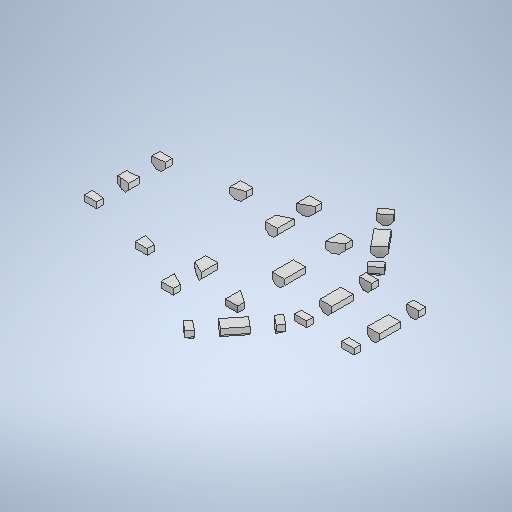
# Autodesk Inventor part: RR_SingleTurnout_Pillow
Saved by Autodesk Inventor 2025.1 (Build 291241000, 241)
## iProperties
Created: 2025-03-08
Part Number: RR_SingleTurnout_Pillow
Material: 一般
Document SubType Name: Modeling
Designer: kumagai
Density: 1 g/cm^3
Appearance: 既定
Author: kumagai
Autodesk Inventor part; units mm, degrees
ref_plane "YZ Plane" through (0, 0, 0) normal (1, 0, 0) x (0, 1, 0)
ref_plane "XZ Plane" through (0, 0, 0) normal (0, 1, 0) x (-1, 0, 0)
ref_plane "XY Plane" through (0, 0, 0) normal (0, 0, 1) x (1, 0, 0)
derived "RR_ThreeWay.ipt"
sketch "MainSketch" plane through (0, 0, 0) normal (0, 1, 0) x (-1, 0, 0)
  line L0 (0, -344.2613) -> (0, 286.2613)
  line L1 (-272.9287, 0) -> (62.5724, 0)
  line L2 (14.6437, -29) -> (-5, -29)
  line L3 (-5, -49.5106) -> (-5, -5.6416)
  line L4 (-5, -48) -> (0, -48)
  line L5 (-5, -10) -> (0, -10)
  line L6 (-5, -38.3) -> (0, -38.3)
  line L7 (-5, -19.7) -> (0, -19.7)
  line L8 (-5, -46) -> (0, -46)
  line L9 (-5, -35.9) -> (0, -35.9)
  line L10 (-5, -22.1) -> (0, -22.1)
  line L11 (-5, -12) -> (0, -12)
  line L12 (-10, -10) -> (-10, -29)
  line L13 (-225, -48) -> (-225, -29)
  line L14 (-120.9077, -19.7) -> (-225, -19.7)
  arc A0 (-10, -48) -> (-148.5929, -105.4071) centre (-10, -244) ccw
  arc A1 (-10, -46) -> (-150.0071, -103.9929) centre (-10, -244) ccw
  line L15 (-143.2215, -110.7785) -> (-189.5102, -64.4898)
  line L16 (-210, -35.9) -> (-210, -29)
  line L17 (-146.1596, -86.6272) -> (-155.9415, -76.8453)
  arc A2 (-133.8847, -47.8455) -> (-174.0488, -79.9512) centre (-10, -244) ccw
  arc A3 (-139.2229, -48.9168) -> (-175.463, -78.537) centre (-10, -244) ccw
  line L18 (-139.499, -48) -> (-225, -48)
  line L19 (-134.4186, -46) -> (-225, -46)
  arc A4 (-118.9103, -50.6657) -> (-166.907, -87.093) centre (-10, -244) ccw
  arc A5 (-120.0882, -48.5746) -> (-168.6041, -85.3959) centre (-10, -244) ccw
  line L20 (-94.2219, -46) -> (-110.2721, -46)
  arc A6 (-111.9271, -35.5897) -> (-114.1724, -36.7028) centre (-10, -244) ccw
  line L21 (-120.9077, -35.9) -> (-225, -35.9)
  line L22 (-120.9077, -38.3) -> (-225, -38.3)
  arc A7 (-133.8847, -47.8455) -> (-134.4186, -46) centre (-134.4186, -47) ccw
  arc A8 (-139.2229, -48.9168) -> (-139.499, -48) centre (-139.499, -48.5) ccw
  arc A9 (-110.2721, -48.4) -> (-118.9103, -50.6657) centre (-110.2721, -66) ccw
  arc A10 (-110.2721, -46) -> (-120.0882, -48.5746) centre (-110.2721, -66) ccw
  arc A11 (-120.9077, -38.3) -> (-114.1724, -36.7028) centre (-120.9077, -23.3) ccw
  arc A12 (-120.9077, -35.9) -> (-115.25, -34.5584) centre (-120.9077, -23.3) ccw
  arc A13 (-143.5264, -51.2283) -> (-148.5252, -54.7884) centre (-10, -244) ccw
  arc A14 (-112.9815, -33.4337) -> (-115.25, -34.5584) centre (-10, -244) ccw
  line L23 (-120.9077, -22.1) -> (-225, -22.1)
  circle A15 centre (-86.125, -22.2) radius 2.5
  arc A16 (-96.415, -52.9331) -> (-105.3417, -57.2273) centre (-10, -244) ccw
  arc A17 (-96.4922, -49.4759) -> (-95.7188, -53.2122) centre (-89.6121, -50) ccw
  arc A18 (-93.3838, -47.5455) -> (-92.1285, -53.7307) centre (-89.6121, -50) ccw
  arc A19 (-96.1897, -54.5879) -> (-157.1489, -96.8511) centre (-10, -244) ccw
  line L24 (-97.4893, -48.4) -> (-110.2721, -48.4)
  arc A20 (-92.2877, -55.4762) -> (-155.4519, -98.5481) centre (-10, -244) ccw
  arc A21 (-92.2877, -55.4762) -> (-92.1285, -53.7307) centre (-92.6877, -54.5597) ccw
  arc A22 (-93.3838, -47.5455) -> (-94.2219, -46) centre (-94.2219, -47) ccw
  arc A23 (-96.1897, -54.5879) -> (-95.7188, -53.2122) centre (-96.6039, -53.6777) ccw
  arc A24 (-96.4922, -49.4759) -> (-97.4893, -48.4) centre (-97.4893, -49.4) ccw
  circle A25 centre (-89.6121, -50) radius 2.5
  line L25 (-42.4799, -17.7596) -> (-25.8571, -19.9879)
  arc A26 (-25.9153, -20.5847) -> (-85.6348, -24.6515) centre (-40.1446, -252.1479) ccw
  arc A27 (-85.7928, -19.7222) -> (-85.6348, -24.6515) centre (-86.125, -22.2) ccw
  arc A28 (-25.9153, -20.5847) -> (-25.8571, -19.9879) centre (-25.8969, -20.2853) ccw
  arc A29 (-42.4799, -17.7596) -> (-76.3848, -20.5664) centre (-40.1446, -252.1479) ccw
  line L26 (-85.7928, -19.7222) -> (-79.2595, -20.598)
  arc A30 (-79.2595, -20.598) -> (-76.3848, -20.5664) centre (-77.9308, -10.6866) ccw
  circle A31 centre (-89.6121, -50) radius 4
  line L27 (-89.754, -46.0025) -> (-25.5965, -43.7259)
  arc A32 (-25.552, -44.3238) -> (-40.8225, -46.6677) centre (-3.1703, -241.0547) ccw
  arc A33 (-25.552, -44.3238) -> (-25.5965, -43.7259) centre (-25.5859, -44.0257) ccw
  arc A34 (-74.4895, -48.1141) -> (-87.9633, -53.6443) centre (-3.1703, -241.0547) ccw
  line L28 (-72.9332, -47.8071) -> (-40.8225, -46.6677)
  arc A35 (-72.9332, -47.8071) -> (-74.4895, -48.1141) centre (-72.7559, -52.804) ccw
  arc A36 (-44.0479, -18.9806) -> (-84.6326, -23.2308) centre (-40.1446, -252.1479) ccw
  arc A37 (-27.9859, -39.0878) -> (-44.4613, -41.2072) centre (-10, -244) ccw
  line L29 (-31.1334, -19.7) -> (-47.6548, -19.7)
  arc A38 (-10, -22.1) -> (-22.0271, -22.4262) centre (-10, -244) ccw
  arc A39 (-44.7432, -24.8368) -> (-62.9678, -28.5145) centre (-10, -244) ccw
  arc A40 (-10, -19.7) -> (-22.1572, -20.0297) centre (-10, -244) ccw
  arc A41 (-45.119, -22.4664) -> (-72.2793, -28.5197) centre (-10, -244) ccw
  arc A42 (-25.457, -23.6967) -> (-43.178, -22.3501) centre (-51.8841, -254.1867) ccw
  line L30 (-24.9, -22.9254) -> (-24.9, -23.2)
  arc A43 (-25.457, -23.6967) -> (-24.9, -23.2) centre (-25.4, -23.2) ccw
  arc A44 (-22.1572, -20.0297) -> (-24.9, -22.9254) centre (-22, -22.9254) ccw
  arc A45 (-43.178, -22.3501) -> (-45.119, -22.4664) centre (-43.5532, -32.343) ccw
  arc A46 (-25.7303, -26.0811) -> (-43.268, -24.7484) centre (-51.8841, -254.1867) ccw
  arc A47 (-22.0271, -22.4262) -> (-22.5, -22.9254) centre (-22, -22.9254) ccw
  line L31 (-22.5, -22.9254) -> (-22.5, -23.2)
  arc A48 (-25.7303, -26.0811) -> (-22.5, -23.2) centre (-25.4, -23.2) ccw
  arc A49 (-43.268, -24.7484) -> (-44.7432, -24.8368) centre (-43.5532, -32.343) ccw
  line L32 (-55.2, -53.283) -> (-55.2, -10)
  line L33 (-40.8, -50.4351) -> (-40.8, -10)
  line L34 (-48, 3.552) -> (-48, 5.2256)
  line L35 (-59, -61.5) -> (-37, -61.5)
  line L36 (-40.8, -10) -> (-40.8, -7.4996)
  line L37 (-55.2, -10) -> (-55.2, -7.4996)
  line L38 (-48, -61.9179) -> (-48, -64.1825)
  line L39 (-37, -61.5) -> (-37, -70.5)
  line L40 (-40, -73.5) -> (-42, -73.5)
  line L41 (-42, -73.5) -> (-40, -62)
  line L42 (-40, -62) -> (-56, -62)
  line L43 (-56, -62) -> (-54, -73.5)
  line L44 (-54, -73.5) -> (-56, -73.5)
  line L45 (-59, -70.5) -> (-59, -58.1371)
  arc A50 (-40, -73.5) -> (-37, -70.5) centre (-40, -70.5) ccw
  arc A51 (-59, -70.5) -> (-56, -73.5) centre (-56, -70.5) ccw
  line L46 (-37, -61.5) -> (-37, -49.8686)
  line L47 (-40.8, -50.4351) -> (-40.8, -62)
  line L48 (-55.2, -53.283) -> (-55.2, -62)
  arc A52 (-34.3731, -49.5213) -> (-37, -52.498) centre (-34, -52.498) ccw
  arc A53 (-59, -58.1371) -> (-62.8083, -55.2481) centre (-62, -58.1371) ccw
  line L49 (-10, -29) -> (-225, -29)
  arc A54 (-151.7465, 120.5538) -> (-11.4945, 29.8813) centre (-10, 186) ccw
  arc A55 (-22.0271, -35.5738) -> (-10, -35.9) centre (-10, 186) ccw
  arc A56 (-22.1572, -37.9703) -> (-10, -38.3) centre (-10, 186) ccw
  arc A57 (-43.268, -33.2516) -> (-25.7303, -31.9189) centre (-51.8841, 196.1867) ccw
  arc A58 (-43.178, -35.6499) -> (-25.457, -34.3033) centre (-51.8841, 196.1867) ccw
  arc A59 (-62.9678, -29.4855) -> (-44.7432, -33.1632) centre (-10, 186) ccw
  arc A60 (-72.2793, -29.4803) -> (-45.119, -35.5336) centre (-10, 186) ccw
  arc A61 (-45.119, -35.5336) -> (-43.178, -35.6499) centre (-43.5532, -25.657) ccw
  arc A62 (-44.7432, -33.1632) -> (-43.268, -33.2516) centre (-43.5532, -25.657) ccw
  arc A63 (-22.5, -35.0746) -> (-22.0271, -35.5738) centre (-22, -35.0746) ccw
  arc A64 (-24.9, -35.0746) -> (-22.1572, -37.9703) centre (-22, -35.0746) ccw
  line L50 (-24.9, -35.0746) -> (-24.9, -34.8)
  line L51 (-22.5, -35.0746) -> (-22.5, -34.8)
  arc A65 (-24.9, -34.8) -> (-25.457, -34.3033) centre (-25.4, -34.8) ccw
  arc A66 (-22.5, -34.8) -> (-25.7303, -31.9189) centre (-25.4, -34.8) ccw
  arc A67 (-62.9678, -28.5145) -> (-63.3485, -29) centre (-62.8485, -29) ccw
  arc A68 (-72.2793, -28.5197) -> (-72.6405, -29) centre (-72.1405, -29) ccw
  arc A69 (-108.1902, -15.666) -> (-89.3785, -23.7845) centre (-10, 186) ccw
  arc A70 (-91.0057, 5.3288) -> (-16.6975, -11.8867) centre (-10, 186) ccw
  arc A71 (-122.8924, 131.193) -> (-43.8763, 65.1658) centre (-10, 186) ccw
  arc A72 (-148.5252, -3.2116) -> (-143.5264, -6.7717) centre (-10, 186) ccw
  circle A73 centre (-86.125, -35.8) radius 2.5
  arc A74 (-85.7286, -33.3316) -> (-25.8975, -35.1189) centre (-48.9436, 195.7336) ccw
  line L52 (-25.8166, -35.7131) -> (-42.3424, -38.5735)
  arc A75 (-25.8166, -35.7131) -> (-25.8975, -35.1189) centre (-25.8677, -35.4174) ccw
  line L53 (-85.6986, -38.2634) -> (-79.2034, -37.1391)
  arc A76 (-76.3296, -37.0611) -> (-79.2034, -37.1391) centre (-77.4979, -46.9926) ccw
  arc A77 (-76.3296, -37.0611) -> (-42.3424, -38.5735) centre (-48.9436, 195.7336) ccw
  arc A78 (-49.1227, -37.4664) -> (-46.0444, -37.4484) centre (-48.9436, 195.7336) ccw
  line L54 (-86.4807, -38.2746) -> (-94.1197, -37.1765)
  arc A79 (-94.2268, -36.2144) -> (-94.1197, -37.1765) centre (-94.0486, -36.6816) ccw
  line L55 (-87.0159, -33.4641) -> (-94.2268, -36.2144)
  line L56 (-76.4926, -34.8148) -> (-77.6457, -34.6296)
  arc A80 (-96.055, -36.8647) -> (-107.6082, -42.0517) centre (-10, -244) ccw
  circle A81 centre (-89.6121, -8) radius 4
  line L57 (-89.6178, -12) -> (-25.42, -12.0915)
  arc A82 (-88.0883, -4.3016) -> (-74.4341, -9.37) centre (-9.7235, 185.8863) ccw
  arc A83 (-74.4341, -9.37) -> (-72.8683, -9.6239) centre (-72.8611, -4.6239) ccw
  line L58 (-72.8683, -9.6239) -> (-40.7373, -9.6697)
  arc A84 (-40.7373, -9.6697) -> (-25.3959, -11.4925) centre (-9.7235, 185.8863) ccw
  arc A85 (-25.42, -12.0915) -> (-25.3959, -11.4925) centre (-25.4196, -11.7915) ccw
  line L59 (-41.4, -73.5) -> (-41.4, -70.05)
  line L60 (-54.6, -73.5) -> (-54.6, -70.05)
  line L61 (-21.7393, -64.7371) -> (-21.7393, -55.7371)
  line L62 (-51.6, 5.7033) -> (-51.6, 3.6437)
  line L63 (-44.4, 6.6538) -> (-44.4, 3.6437)
  line L64 (-44.4, -63.9796) -> (-44.4, -61.3243)
  line L65 (-51.6, -63.5159) -> (-51.6, -61.3243)
  arc A86 (-106.8215, -31.0506) -> (-105.9722, -29) centre (-108.8722, -29) ccw
  arc A87 (-111.9271, -35.5897) -> (-109.9456, -34.1747) centre (-115.1782, -28.9421) ccw
  line L66 (-109.9456, -34.1747) -> (-106.8215, -31.0506)
  arc A88 (-112.9815, -33.4337) -> (-111.6427, -32.4776) centre (-115.1782, -28.9421) ccw
  arc A89 (-108.5186, -29.3536) -> (-108.3722, -29) centre (-108.8722, -29) ccw
  line L67 (-111.6427, -32.4776) -> (-108.5186, -29.3536)
  arc A90 (-63.3485, -29) -> (-62.9678, -29.4855) centre (-62.8485, -29) ccw
  arc A91 (-72.6405, -29) -> (-72.2793, -29.4803) centre (-72.1405, -29) ccw
  line L68 (-210, -29) -> (-210, -22.1)
  line L69 (-225, -29) -> (-225, -10)
  line L70 (-10, -29) -> (-10, -48)
  line L71 (-22.0231, -12) -> (-39.3668, -12)
  line L72 (-157.1489, -96.8511) -> (-146.5423, -86.2445)
  point P0 (0, 0)
  point P1 (-90.8602, -19.7)
  point P2 (-94.9346, -22.1)
  point P3 (-96.3241, -48.4)
  point P4 (-87.5506, -46)
  point P5 (-162.028, -91.972)
  point P6 (-44.0258, -45.5806)
  point P7 (-48, -2.9806)
  point P8 (-48, -61.5806)
  point P9 (-37, -73.5)
  point P10 (-59, -73.5)
  point P11 (-51.2642, -37.4549)
  point P12 (-51.1178, -10.8549)
  point P13 (-103.3722, -29)
  point P14 (-48, -53.4549)
sketch "PillowSketch" plane through (0, 0, 0) normal (0, 1, 0) x (-1, 0, 0)
  line L0 (-40, -1.4534) -> (-40, 7.7945)
  line L1 (-71, -1.7421) -> (-71, 3.0229)
  line L2 (-102, -0.653) -> (-102, 5.4734)
  line L3 (-133, -1.0497) -> (-133, 3.4642)
  line L4 (-164, -2.8834) -> (-164, 3.4642)
  line L5 (-195, -2.8121) -> (-195, 3.534)
  line L6 (-121.4315, -106.3936) -> (-109.7227, -120.8528)
  line L7 (-101.8172, -89.6691) -> (-92.4243, -105.4573)
  line L8 (-79.3942, -76.4675) -> (-71.1859, -96.2843)
  line L9 (-75, -63.4919) -> (-67, -63.4919)
  line L10 (-106, -77.5199) -> (-98, -77.5199)
  line L11 (-156.8999, -56.2377) -> (-163.117, -61.2723)
  line L12 (-133.6607, -97.6478) -> (-127.4435, -92.6133)
  line L13 (-137, -66.4368) -> (-129, -66.4368)
  line L14 (-168, -52.4) -> (-160, -52.4)
  line L15 (-199, -52.4) -> (-191, -52.4)
  line L16 (-160, -52.4) -> (-160, -48)
  line L17 (-168, -48) -> (-168, -52.4)
  line L18 (-191, -52.4) -> (-191, -48)
  line L19 (-199, -48) -> (-199, -52.4)
  line L20 (-137, -62.0368) -> (-137, -66.4368)
  line L21 (-129, -66.4368) -> (-129, -56.7072)
  line L22 (-98, -77.5199) -> (-98, -68.8658)
  line L23 (-98, -55.4221) -> (-98, -48.4)
  line L24 (-106, -48.4) -> (-106, -59.3663)
  line L25 (-106, -73.1199) -> (-106, -77.5199)
  line L26 (-67, -63.4919) -> (-67, -56.4713)
  line L27 (-75, -59.0919) -> (-75, -63.4919)
  line L28 (-28, -2.7496) -> (-28, 7.3369)
  line L29 (-32, -53.6386) -> (-24, -53.6386)
  line L30 (-24, -53.6386) -> (-24, -48.5006)
  line L31 (-32, -49.2386) -> (-32, -53.6386)
  line L32 (-136.4297, -94.2284) -> (-133.6607, -97.6478)
  line L33 (-127.4435, -92.6133) -> (-130.2125, -89.1938)
  line L34 (-163.117, -61.2723) -> (-160.348, -64.6917)
  line L35 (-152.7321, -74.0966) -> (-144.046, -84.8231)
  line L36 (-137.8288, -79.7885) -> (-146.5149, -69.062)
  line L37 (-154.1309, -59.6571) -> (-156.8999, -56.2377)
  line L38 (-143.2215, -110.7785) -> (-189.5102, -64.4898) projected
  arc A0 (-10, -48) -> (-148.5929, -105.4071) centre (-10, -244) ccw projected
  arc A1 (-139.2229, -48.9168) -> (-175.463, -78.537) centre (-10, -244) ccw projected
  arc A2 (-96.1897, -54.5879) -> (-157.1489, -96.8511) centre (-10, -244) ccw projected
  arc A3 (-118.9103, -50.6657) -> (-166.907, -87.093) centre (-10, -244) ccw projected
  line L39 (-97.4893, -48.4) -> (-110.2721, -48.4) projected
  line L40 (-10, -29) -> (-225, -29) projected
  line L41 (-120.9077, -35.9) -> (-225, -35.9) projected
  line L42 (-225, -48) -> (-225, -29) projected
  line L43 (-10, -29) -> (-10, -48) projected
  line L44 (-139.499, -48) -> (-225, -48) projected
  line L45 (-160, -35.9) -> (-160, -29)
  line L46 (-168, -35.9) -> (-168, -29)
  line L47 (-191, -35.9) -> (-191, -29)
  line L48 (-199, -35.9) -> (-199, -29)
  arc A4 (-43.268, -33.2516) -> (-25.7303, -31.9189) centre (-51.8841, 196.1867) ccw projected
  arc A5 (-22.5, -34.8) -> (-25.7303, -31.9189) centre (-25.4, -34.8) ccw projected
  arc A6 (-25.7303, -26.0811) -> (-22.5, -23.2) centre (-25.4, -23.2) ccw projected
  arc A7 (-25.7303, -26.0811) -> (-43.268, -24.7484) centre (-51.8841, -254.1867) ccw projected
  line L49 (-32, -32.5507) -> (-32, -29)
  line L50 (-24, -32.6357) -> (-24, -29)
  line L51 (-129, -35.9) -> (-129, -29)
  line L52 (-137, -35.9) -> (-137, -29)
  point P0 (0, 0)
  point P1 (-24, -32.2603)
  dimension "d2" = 31
  dimension "d3" = 31
  dimension "d4" = 31
  dimension "d5" = 31
  dimension "d6" = 31
  dimension "d9" = 8.25
  dimension "d10" = 8.25
  dimension "d17" = 4.4
  dimension "d19" = 4.4
  dimension "d21" = 4.4
  dimension "d25" = 4.4
  dimension "d27" = 8
  dimension "d28" = 4.4
  dimension "d29" = 4.4
  dimension "d38" = 30
  dimension "d39" = 30
  dimension "d40" = 18
  dimension "d41" = 6
  dimension "d42" = 8
  dimension "d43" = 8
  dimension "d44" = 8
  dimension "d45" = 8
  dimension "d46" = 8
  dimension "d47" = 8
  dimension "d48" = 4.4
  constraints: 92 end point, 16 point on line, 15 collinear, 11 point on circle, 6 perpendicular, 6 vertical, 4 horizontal, 3 parallel, 25 other
  measures "d2" distance between parallel lines of L4 L5
  measures "d3" distance between parallel lines of L3 L4
  measures "d4" distance between parallel lines of L2 L3
  measures "d5" distance between parallel lines of L2 L1
  measures "d6" distance between parallel lines of L0 L1
  measures "d9" angle of L7 L6
  measures "d10" angle of L8 L7
  measures "d17" distance of L20.start L13.start
  measures "d19" distance of L25.start L10.start
  measures "d21" distance of L27.start L9.start
  measures "d25" distance of L29.start L31.start
  measures "d27" distance between parallel lines of L33 L32
  measures "d28" distance of L32.start L12.start
  measures "d29" distance of L11.end L34.end
  measures "d38" distance between parallel lines of L5 L42
  measures "d39" distance between parallel lines of L0 L43
  measures "d40" distance between parallel lines of L28 L43
  measures "d41" angle of L38 L6
  measures "d42" distance between parallel lines of L31 L30
  measures "d43" distance between parallel lines of L27 L26
  measures "d44" distance between parallel lines of L25 L22
  measures "d45" distance between parallel lines of L20 L21
  measures "d46" distance between parallel lines of L17 L16
  measures "d47" distance between parallel lines of L19 L18
  measures "d48" distance between parallel lines of L44 L14
extrude "PillowBody" add sketch "PillowSketch" along normal blind 2.1 and the other way blind 4.2 contours L27 A0 L26 L9 | L25 A0 L22 L10 | L37 A1 L34 L11 | L32 A0 L33 L12 | L20 A3 L21 L13 | L17 L44 L16 L14 | L19 L44 L18 L15 | A2 L24 L39 L23 | L31 A0 L30 L29 | A3 L36 A2 L35 | L50 A5 A4 L49 L40 | L51 L41 L52 L40 | L45 L41 L46 L40 | L47 L41 L48 L40
chamfer "PillowChamfer" distance 2.5 angle 45 36 edges at (24, -4.2, -51.0696) (28, -4.2, -53.6386) (32, -4.2, -51.4386) (75, -4.2, -61.2919) (67, -4.2, -59.9816) (71, -4.2, -63.4919) (102, -4.2, -77.5199) (106, -4.2, -75.3199) (98, -4.2, -73.1928) (98, -4.2, -51.9111) (106, -4.2, -53.8831) (129, -4.2, -61.572) (133, -4.2, -66.4368) (137, -4.2, -64.2368) (142.1719, -4.2, -74.4253) (148.389, -4.2, -79.4598) (135.0452, -4.2, -95.9381) (128.828, -4.2, -90.9036) (130.5521, -4.2, -95.1306) (164, -4.2, -52.4) (168, -4.2, -50.2) (160, -4.2, -50.2) (199, -4.2, -50.2) (195, -4.2, -52.4) (191, -4.2, -50.2) (32, -4.2, -30.7753) (24, -4.2, -30.6302) (160, -4.2, -32.45) (168, -4.2, -32.45) (191, -4.2, -32.45) (199, -4.2, -32.45) (137, -4.2, -32.45) (129, -4.2, -32.45) (161.7325, -4.2, -62.982) (155.5154, -4.2, -57.9474) (160.0085, -4.2, -58.755)
mirror "ミラー1" about plane through (129, 0, -29) normal (0, 0, 1)
